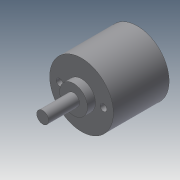
# Autodesk Inventor part: Gantry Motor
Saved by Autodesk Inventor 2014 SP1 (Build 180222100, 222)
## iProperties
Created: 2014-04-10
Part Number: Gantry Motor
Material: Generic
Document SubType Name: Modeling
Designer: tom
Density: 1 g/cm^3
Appearance: Brass - Satin
Author: tom
Autodesk Inventor part; units mm, degrees
ref_plane "YZ Plane" through (0, 0, 0) normal (1, 0, 0) x (0, 1, 0)
ref_plane "XZ Plane" through (0, 0, 0) normal (0, 1, 0) x (-1, 0, 0)
ref_plane "XY Plane" through (0, 0, 0) normal (0, 0, 1) x (1, 0, 0)
sketch "Sketch1" plane through (0, 0, 0) normal (0, 0, 1) x (1, 0, 0)
  circle A0 centre (0, 0) radius 8
  dimension "d0" = 16
  constraints: 1 centre point, 1 coincident
  measures "d0" diameter of A0
extrude "Extrusion1" add sketch "Sketch1" along normal blind 14
sketch "Sketch2" plane through (0, 0, 14) normal (0, 0, 1) x (1, 0, 0)
  circle A0 centre (0, 0) radius 8 projected
  circle A1 centre (5.5, 0) radius 0.85
  circle A2 centre (-5.5, 0) radius 0.85
  dimension "d3" = 1.7
  dimension "d4" = 1.7
  dimension "d5" = 5.5
  dimension "d6" = 5.5
  constraints: 2 centre point
  measures "d3" diameter of A1
  measures "d4" diameter of A2
  measures "d5" distance of A0.centre A2.centre
  measures "d6" distance of A0.centre A1.centre
extrude "Extrusion2" cut sketch "Sketch2" against normal blind 10 contours A1 | A2
sketch "Sketch3" plane through (0, 0, 14) normal (0, 0, 1) x (1, 0, 0)
  circle A0 centre (0, 0) radius 8 projected
  circle A1 centre (0, 0) radius 3.5
  dimension "d9" = 7
  constraints: 1 centre point, 1 coincident
  measures "d9" diameter of A1
extrude "Extrusion3" add sketch "Sketch3" along normal blind 2 contours A1
sketch "Sketch4" plane through (0, 0, 16) normal (0, 0, 1) x (1, 0, 0)
  circle A0 centre (0, 0) radius 3.5 projected
  circle A1 centre (0, 0) radius 1.5
  dimension "d12" = 3
  constraints: 1 centre point, 1 coincident
  measures "d12" diameter of A1
extrude "Extrusion4" add sketch "Sketch4" along normal blind 7.75 contours A1
sketch "Sketch5" plane through (0, 0, 0) normal (0, 0, -1) x (-1, 0, 0)
  circle A0 centre (0, 0) radius 8 projected
  line L0 (-4.8302, 5.9) -> (4.8302, 5.9)
  line L1 (-4.8302, -5.9) -> (4.8302, -5.9)
  arc A1 (-4.8302, 5.9) -> (-4.8302, -5.9) centre (0, 0) ccw
  arc A2 (4.8302, -5.9) -> (4.8302, 5.9) centre (0, 0) ccw
  dimension "d16" = 5.9
  dimension "d17" = 5.9
  constraints: 4 end point, 4 point on circle, 2 centre point, 1 coincident, 1 horizontal, 1 parallel
  measures "d16" distance from line of L0 A1.centre
  measures "d17" distance from line of A0.centre L1
extrude "Extrusion5" add sketch "Sketch5" along normal blind 18.4 contours L0 A2 L1 A1
fillet "Fillet1" radius 0.5 4 edges at (0, 5.9, -18.4) (7.625, 0, -18.4) (-7.625, 0, -18.4) (0, -5.9, -18.4)
sketch "Sketch6" plane through (0, 0, -18.4) normal (0, 0, -1) x (-1, 0, 0)
  arc A0 (-4.6482, 5.4) -> (-4.6482, -5.4) centre (0, 0) ccw projected
  circle A1 centre (0, 0) radius 2.5
  dimension "d21" = 5
  constraints: 1 centre point, 1 coincident
  measures "d21" diameter of A1
extrude "Extrusion6" add sketch "Sketch6" along normal blind 0.5
body "Solid1"
